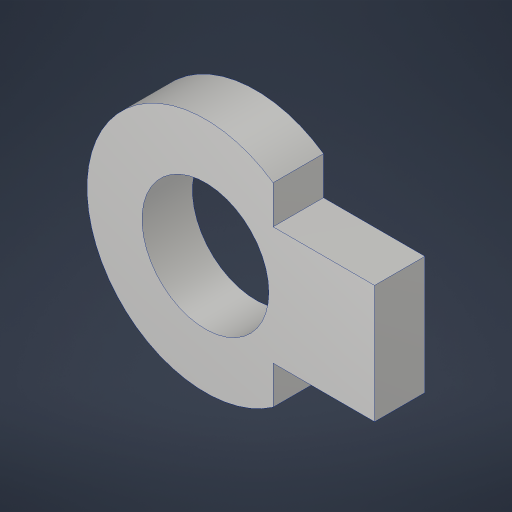
# Autodesk Inventor part: EL2-A-009
Saved by Autodesk Inventor 2023.4 (Build 274418000, 418)
## iProperties
Created: 2025-01-21
Part Number: EL2-A-009
Material: Aluminum 6061
Document SubType Name: Modeling
Designer: brand
Density: 2.7 g/cm^3
Appearance: Aluminum - Flat
Author: brand
Autodesk Inventor part; units mm, degrees
ref_plane "YZ Plane" through (0, 0, 0) normal (1, 0, 0) x (0, 1, 0)
ref_plane "XZ Plane" through (0, 0, 0) normal (0, 1, 0) x (-1, 0, 0)
ref_plane "XY Plane" through (0, 0, 0) normal (0, 0, 1) x (1, 0, 0)
sketch "Sketch1" plane through (0, 0, 0) normal (0, 0, 1) x (1, 0, 0)
  circle A0 centre (0, 0) radius 23.8125
  circle A1 centre (0, 0) radius 44.45 construction
  line L0 (25.4, 22.1615) -> (63.5, 22.1615)
  line L1 (63.5, 22.1615) -> (63.5, -22.1615)
  line L2 (63.5, -22.1615) -> (25.4, -22.1615)
  arc A2 (25.4, 36.478) -> (25.4, -36.478) centre (0, 0) ccw
  line L3 (25.4, 36.478) -> (25.4, 22.1615)
  line L4 (25.4, -36.478) -> (25.4, -22.1615)
  point P0 (63.5, 0)
  dimension "d1" = 88.9
  dimension "d0" = 47.625
  dimension "d2" = 44.323
  dimension "d3" = 38.1
  dimension "d4" = 25.4
  constraints: 10 end point, 3 coincident, 3 point on circle, 2 centre point, 2 perpendicular, 2 vertical, 1 horizontal, 1 horizontal alignment, 1 midpoint, 1 vertical alignment, 3 other
  measures "d0" diameter of A0
  measures "d2" distance of L0.end L1.end
  measures "d3" distance of L0.start L0.end
  measures "d4" distance from line of point (0, 0) L3
extrude "Extrusion1" add sketch "Sketch1" along normal mid plane 18.923
body "Solid1"
